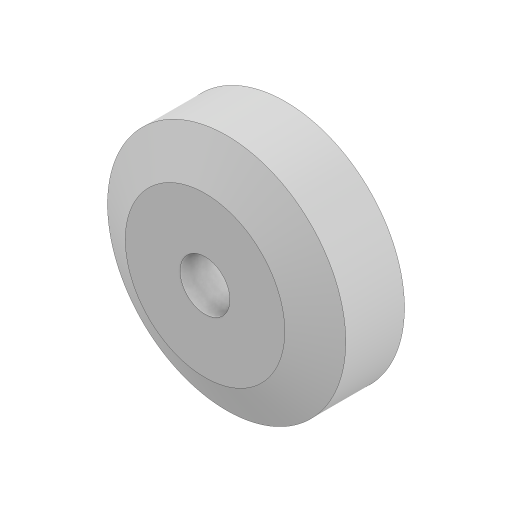
# Autodesk Inventor part: RUEDA
Saved by Autodesk Inventor 2024 (Build 280153000, 153)
## iProperties
Created: 2024-05-16
Part Number: RUEDA
Material: Generic
Document SubType Name: Modeling
Designer: Jhuliams
Density: 1 g/cm^3
Appearance: Default
Author: Jhuliams
Autodesk Inventor part; units mm, degrees
ref_plane "YZ Plane" through (0, 0, 0) normal (1, 0, 0) x (0, 1, 0)
sketch "Sketch1" plane through (0, 0, 0) normal (0, 0, 1) x (1, 0, 0)
  circle A0 centre (0, -0.3986) radius 11.95
  point P0 (0, 0)
  dimension "d0" = 23.9
  constraints: 1 centre point
  measures "d0" diameter of A0
extrude "Extrusion1" add sketch "Sketch1" along normal blind 5.89
ref_plane "Work Plane1" through (0, -0.3986, 8.06) normal (0, 0, 1) x (1, 0, 0)
sketch "Sketch2" plane through (0, -0.3986, 8.06) normal (0, 0, 1) x (1, 0, 0)
  circle A0 centre (0, 0) radius 8
  point P0 (0, 0.3986)
  dimension "d4" = 16
  constraints: 1 centre point
  measures "d4" diameter of A0
sketch "Sketch5" plane through (0, -0.3986, 5.89) normal (0, 0, 1) x (1, 0, 0)
  circle A0 centre (0, 0) radius 11.95
  point P0 (0, 0.3986)
  dimension "d5" = 23.9
  constraints: 1 centre point
  measures "d5" diameter of A0
loft "Loft1" add profiles "Sketch2", "Sketch5"
ref_plane "Work Plane2" through (0, -0.3986, -2.17) normal (0, 0, -1) x (-1, 0, 0)
sketch "Sketch6" plane through (0, -0.3986, -2.17) normal (0, 0, -1) x (-1, 0, 0)
  circle A0 centre (0, 0) radius 8
  point P0 (0, 0.3986)
  dimension "d11" = 16
  constraints: 1 centre point
  measures "d11" diameter of A0
sketch "Sketch7" plane through (0, -0.3986, 0) normal (0, 0, -1) x (-1, 0, 0)
  circle A0 centre (0, 0) radius 11.95
  point P0 (0, 0.3986)
  dimension "d12" = 23.9
  constraints: 1 centre point
  measures "d12" diameter of A0
loft "Loft2" add profiles "Sketch6", "Sketch7"
sketch "Sketch8" plane through (0, -0.3986, 8.06) normal (0, 0, 1) x (1, 0, 0)
  circle A0 centre (0, 0) radius 2.5
  point P0 (0, 0.3986)
  dimension "d17" = 5
  constraints: 1 centre point
  measures "d17" diameter of A0
extrude "Extrusion2" cut sketch "Sketch8" against normal blind 15
body "Solid1"
